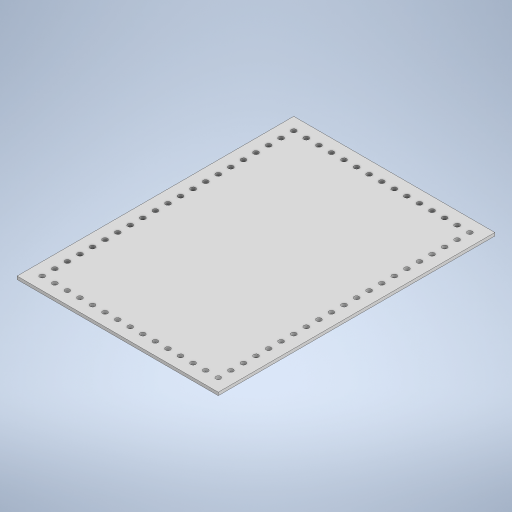
# Autodesk Inventor part: Top Plate
Saved by Autodesk Inventor 2023.4 (Build 274418000, 418)
## iProperties
Created: 2023-12-24
Part Number: Top Plate
Material: Generic
Document SubType Name: Sheet Metal
Designer: amrom
Density: 1 g/cm^3
Sheet Metal Rule: Default
Appearance: Default
Author: amrom
Autodesk Inventor part; units mm, degrees
ref_plane "YZ Plane" through (0, 0, 0) normal (1, 0, 0) x (0, 1, 0)
ref_plane "XZ Plane" through (0, 0, 0) normal (0, 1, 0) x (-1, 0, 0)
ref_plane "XY Plane" through (0, 0, 0) normal (0, 0, 1) x (1, 0, 0)
sketch "Sketch1" plane through (0, 0, 0) normal (0, 1, 0) x (-1, 0, 0)
  line L0 (0, 0) -> (203.2, 0)
  line L1 (203.2, 0) -> (203.2, -279.4)
  line L2 (203.2, -279.4) -> (0, -279.4)
  line L3 (0, -279.4) -> (0, 0)
  dimension "d0" = 203.2
  dimension "d1" = 279.4
  measures "d0" distance of L1.end L2.end
  measures "d1" distance of L0.end L1.end
extrude "Plate1" add sketch "Sketch1" along normal blind 3.048
sketch "Sketch2" plane through (0, 3.048, 0) normal (0, 1, 0) x (1, 0, 0)
  circle A0 centre (-12.7, 12.7) radius 2.5019
  line L0 (0, 0) -> (-203.2, 0) projected
  line L1 (0, 279.4) -> (0, 0) projected
  circle A1 centre (-25.4, 12.7) radius 2.5019
  circle A2 centre (-38.1, 12.7) radius 2.5019
  circle A3 centre (-50.8, 12.7) radius 2.5019
  circle A4 centre (-63.5, 12.7) radius 2.5019
  circle A5 centre (-76.2, 12.7) radius 2.5019
  circle A6 centre (-88.9, 12.7) radius 2.5019
  circle A7 centre (-101.6, 12.7) radius 2.5019
  circle A8 centre (-114.3, 12.7) radius 2.5019
  circle A9 centre (-127, 12.7) radius 2.5019
  circle A10 centre (-139.7, 12.7) radius 2.5019
  circle A11 centre (-152.4, 12.7) radius 2.5019
  circle A12 centre (-165.1, 12.7) radius 2.5019
  circle A13 centre (-177.8, 12.7) radius 2.5019
  circle A14 centre (-190.5, 12.7) radius 2.5019
  line L2 (-203.2, 0) -> (-203.2, 279.4) projected
  circle A15 centre (-190.5, 25.4) radius 2.5019
  circle A16 centre (-190.5, 38.1) radius 2.5019
  circle A17 centre (-190.5, 50.8) radius 2.5019
  circle A18 centre (-190.5, 63.5) radius 2.5019
  circle A19 centre (-190.5, 76.2) radius 2.5019
  circle A20 centre (-190.5, 88.9) radius 2.5019
  circle A21 centre (-190.5, 101.6) radius 2.5019
  circle A22 centre (-190.5, 114.3) radius 2.5019
  circle A23 centre (-190.5, 127) radius 2.5019
  circle A24 centre (-190.5, 139.7) radius 2.5019
  circle A25 centre (-190.5, 152.4) radius 2.5019
  circle A26 centre (-190.5, 165.1) radius 2.5019
  circle A27 centre (-190.5, 177.8) radius 2.5019
  circle A28 centre (-190.5, 190.5) radius 2.5019
  circle A29 centre (-190.5, 203.2) radius 2.5019
  circle A30 centre (-190.5, 215.9) radius 2.5019
  circle A31 centre (-190.5, 228.6) radius 2.5019
  circle A32 centre (-190.5, 241.3) radius 2.5019
  circle A33 centre (-190.5, 254) radius 2.5019
  circle A34 centre (-190.5, 266.7) radius 2.5019
  line L3 (-203.2, 279.4) -> (0, 279.4) projected
  circle A35 centre (-177.8, 266.7) radius 2.5019
  circle A36 centre (-165.1, 266.7) radius 2.5019
  circle A37 centre (-152.4, 266.7) radius 2.5019
  circle A38 centre (-139.7, 266.7) radius 2.5019
  circle A39 centre (-127, 266.7) radius 2.5019
  circle A40 centre (-114.3, 266.7) radius 2.5019
  circle A41 centre (-101.6, 266.7) radius 2.5019
  circle A42 centre (-88.9, 266.7) radius 2.5019
  circle A43 centre (-76.2, 266.7) radius 2.5019
  circle A44 centre (-63.5, 266.7) radius 2.5019
  circle A45 centre (-50.8, 266.7) radius 2.5019
  circle A46 centre (-38.1, 266.7) radius 2.5019
  circle A47 centre (-25.4, 266.7) radius 2.5019
  circle A48 centre (-12.7, 266.7) radius 2.5019
  circle A49 centre (-12.7, 254) radius 2.5019
  circle A50 centre (-12.7, 241.3) radius 2.5019
  circle A51 centre (-12.7, 228.6) radius 2.5019
  circle A52 centre (-12.7, 215.9) radius 2.5019
  circle A53 centre (-12.7, 203.2) radius 2.5019
  circle A54 centre (-12.7, 190.5) radius 2.5019
  circle A55 centre (-12.7, 177.8) radius 2.5019
  circle A56 centre (-12.7, 165.1) radius 2.5019
  circle A57 centre (-12.7, 152.4) radius 2.5019
  circle A58 centre (-12.7, 139.7) radius 2.5019
  circle A59 centre (-12.7, 127) radius 2.5019
  circle A60 centre (-12.7, 114.3) radius 2.5019
  circle A61 centre (-12.7, 101.6) radius 2.5019
  circle A62 centre (-12.7, 88.9) radius 2.5019
  circle A63 centre (-12.7, 76.2) radius 2.5019
  circle A64 centre (-12.7, 63.5) radius 2.5019
  circle A65 centre (-12.7, 50.8) radius 2.5019
  circle A66 centre (-12.7, 38.1) radius 2.5019
  circle A67 centre (-12.7, 25.4) radius 2.5019
  dimension "d3" = 5.0038
  dimension "d4" = 12.7
  dimension "d5" = 12.7
  dimension "d8" = 12.7
  dimension "d13" = 5.0038
  dimension "d15" = 12.7
  dimension "d16" = 12.7
  dimension "d19" = 12.7
  dimension "d24" = 5.0038
  dimension "d25" = 12.7
  dimension "d26" = 12.7
  dimension "d29" = 12.7
  dimension "d34" = 5.0038
  dimension "d35" = 12.7
  dimension "d36" = 12.7
  dimension "d39" = 12.7
  constraints: 68 centre point, 2 horizontal, 2 vertical, 128 other
  measures "d3" diameter of A0
  measures "d4" distance from line of L0 A0.centre
  measures "d5" distance from line of L1 A0.centre
  measures "d8" distance of A0.centre A1.centre
  measures "d13" diameter of A14
  measures "d15" distance from line of L2 A14.centre
  measures "d16" distance from line of L0 A14.centre
  measures "d19" distance of A14.centre A15.centre
  measures "d24" diameter of A34
  measures "d25" distance from line of L3 A34.centre
  measures "d26" distance from line of L2 A34.centre
  measures "d29" distance of A34.centre A35.centre
  measures "d34" diameter of A48
  measures "d35" distance from line of L1 A48.centre
  measures "d36" distance from line of L3 A48.centre
  measures "d39" distance of A48.centre A49.centre
extrude "Extrusion1" cut sketch "Sketch2" against normal blind 25.4 contours A0 | A1 | A2 | A3 | A4 | A5 | A6 | A7 | A8 | A9 | A10 | A11 | A12 | A13 | A14 | A15 | A16 | A17 | A18 | A19 | A20 | A21 | A22 | A23 | A24 | A25 | A26 | A27 | A28 | A29 | A30 | A31 | A32 | A33 | A34 | A35 | A36 | A37 | A38 | A39 | A40 | A41 | A42 | A43 | A44 | A45 | A46 | A47 | A48 | A49 | A50 | A51 | A52 | A53 | A54 | A55 | A56 | A57 | A58 | A59 | A60 | A61 | A62 | A63 | A64 | A65 | A66 | A67
equation "\"d2\" = Thickness"
equation "\"BendRadius\" = Thickness"
equation "\"BendReliefWidth\" = Thickness"
equation "\"BendReliefDepth\" = 0.5 * Thickness"
equation "\"CornerReliefSize\" = 4 * Thickness"
equation "\"MinimumRemnant\" = 2 * Thickness"
equation "\"TransitionRadius\" = BendRadius"
equation "\"JacobiRadiusSize\" = BendRadius"
equation "\"GapSize\" = Thickness"
equation "\"Thickness\" = 3.048"
body "Solid1"
